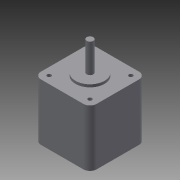
# Autodesk Inventor part: NEMA17
Saved by Autodesk Inventor 2014 (Build 180170000, 170)
## iProperties
Created: 2014-01-09
Part Number: NEMA17
Material: Generic
Document SubType Name: Modeling
Designer: ThatOtherGuy
Density: 1 g/cm^3
Appearance: Default
Author: ThatOtherGuy
Autodesk Inventor part; units mm, degrees
ref_plane "YZ Plane" through (0, 0, 0) normal (1, 0, 0) x (0, 1, 0)
ref_plane "XZ Plane" through (0, 0, 0) normal (0, 1, 0) x (-1, 0, 0)
ref_plane "XY Plane" through (0, 0, 0) normal (0, 0, 1) x (1, 0, 0)
sketch "Sketch1" plane through (0, 0, 0) normal (0, 0, 1) x (1, 0, 0)
  line L0 (5, 0) -> (37.3, 0)
  line L1 (42.3, 5) -> (42.3, 37.3)
  line L2 (37.3, 42.3) -> (5, 42.3)
  line L3 (0, 37.3) -> (0, 5)
  arc A0 (5, 42.3) -> (0, 37.3) centre (5, 37.3) ccw
  arc A1 (42.3, 37.3) -> (37.3, 42.3) centre (37.3, 37.3) ccw
  arc A2 (37.3, 0) -> (42.3, 5) centre (37.3, 5) ccw
  arc A3 (0, 5) -> (5, 0) centre (5, 5) ccw
  point P0 (0, 0)
  dimension "d0" = 42.3
  dimension "d1" = 42.3
  dimension "d2" = 5
  constraints: 8 end point, 8 point on circle, 8 tangent, 4 centre point, 3 equal radius, 2 parallel, 2 point on line, 1 horizontal, 1 perpendicular
  measures "d0" distance between parallel lines of L0 L2
  measures "d1" distance between parallel lines of L1 L3
  measures "d2" radius of A0
extrude "Extrusion1" add sketch "Sketch1" along normal blind 43
sketch "Sketch2" plane through (0, 0, 43) normal (0, 0, 1) x (1, 0, 0)
  line L0 (0, 37.3) -> (0, 5) projected
  line L1 (5, 0) -> (37.3, 0) projected
  line L2 (37.3, 42.3) -> (5, 42.3) projected
  circle A0 centre (5.65, 36.65) radius 1.5
  circle A1 centre (36.65, 36.65) radius 1.5
  circle A2 centre (36.65, 5.65) radius 1.5
  circle A3 centre (5.65, 5.65) radius 1.5
  line L3 (5.65, 5.65) -> (21.15, 21.15)
  line L4 (36.65, 5.65) -> (21.15, 21.15)
  line L5 (21.15, 21.15) -> (36.65, 36.65)
  line L6 (21.15, 21.15) -> (5.65, 36.65)
  line L7 (5.65, 36.65) -> (36.65, 36.65)
  line L8 (5.65, 36.65) -> (5.65, 5.65)
  line L9 (21.15, 21.15) -> (21.15, 0)
  line L10 (0, 21.15) -> (21.15, 21.15)
  point P0 (0, 0)
  dimension "d5" = 31
  dimension "d8" = 3
  dimension "d10" = 21.15
  dimension "d11" = 21.15
  constraints: 16 end point, 6 perpendicular, 4 centre point, 4 equal length, 3 equal radius, 2 midpoint, 1 parallel
  measures "d5" distance of L6.end L5.end
  measures "d8" diameter of A3
  measures "d10" distance of L3.end L9.end
  measures "d11" distance from line of L2 L3.end
extrude "Extrusion2" cut sketch "Sketch2" against normal blind 15 contours L7 L8 A0 | A0 L6 L7 | A2 | L8 L6 A0 | L7 L5 A1 | A1 L5 L7 | L8 L3 A3 | A3 L3 L8
sketch "Sketch3" plane through (0, 0, 43) normal (0, 0, 1) x (1, 0, 0)
  line L0 (0, 37.3) -> (0, 5) projected
  line L1 (5, 0) -> (37.3, 0) projected
  line L2 (37.3, 42.3) -> (5, 42.3) projected
  circle A0 centre (21.15, 21.15) radius 11
  line L3 (0, 21.15) -> (21.15, 21.15)
  line L4 (21.15, 21.15) -> (21.15, 0)
  point P0 (0, 0)
  dimension "d14" = 22
  constraints: 4 end point, 2 midpoint, 1 centre point, 1 parallel, 1 perpendicular
  measures "d14" diameter of A0
extrude "Extrusion3" add sketch "Sketch3" along normal blind 2
sketch "Sketch4" plane through (21.15, 21.15, 45) normal (0, 0, 1) x (1, 0, 0)
  circle A0 centre (0, 0) radius 11 projected
  circle A1 centre (0, 0) radius 2.5
  point P0 (-21.15, -21.15)
  dimension "d19" = 5
  constraints: 1 centre point, 1 coincident
  measures "d19" diameter of A1
extrude "Extrusion4" add sketch "Sketch4" along normal blind 22 contours A1
equation "\"d1\" = d0"
equation "\"d10\" = d11"
body "Solid1"
